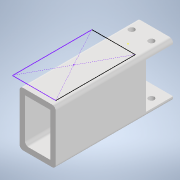
# Autodesk Inventor part: SUCTION_EXTENSION1
Saved by Autodesk Inventor 2021 (Build 250183000, 183)
## iProperties
Created: 2023-03-20
Part Number: SUCTION_EXTENSION1
Material: Generic
Document SubType Name: Modeling
Designer: mahmo
Density: 1 g/cm^3
Appearance: Default
Author: mahmo
Autodesk Inventor part; units mm, degrees
ref_plane "YZ Plane" through (0, 0, 0) normal (1, 0, 0) x (0, 1, 0)
ref_plane "XZ Plane" through (0, 0, 0) normal (0, 1, 0) x (-1, 0, 0)
ref_plane "XY Plane" through (0, 0, 0) normal (0, 0, 1) x (1, 0, 0)
sketch "Sketch1" plane through (0, 0, 0) normal (0, 0, 1) x (1, 0, 0)
  line L0 (-10, 15) -> (10, 15)
  line L1 (10, 15) -> (10, -15)
  line L2 (10, -15) -> (-10, -15)
  line L3 (-10, -15) -> (-10, 15)
  line L4 (-10, 15) -> (10, -15) construction
  line L5 (10, 15) -> (-10, -15) construction
  point P0 (0, 0)
  dimension "d0" = 20
  dimension "d1" = 30
  constraints: 12 end point, 2 midpoint, 2 parallel, 1 horizontal, 1 perpendicular
  measures "d0" distance of L1.end L2.end
  measures "d1" distance of L0.end L1.end
extrude "Extrusion1" add sketch "Sketch1" along normal blind 50
shell "Shell1" thickness 3 removed faces 1 at (-3.3333, 5, 50)
sketch "Sketch2" plane through (-10, 15, 0) normal (0, 1, 0) x (1, 0, 0)
  line L0 (3, -3) -> (17, -3) projected
  line L1 (-7, -47) -> (17, -47)
  line L2 (17, -47) -> (17, -3)
  line L3 (17, -3) -> (-7, -3)
  line L4 (-7, -3) -> (-7, -47)
  line L5 (-7, -47) -> (17, -3) construction
  line L6 (17, -47) -> (-7, -3) construction
  point P0 (10, 0)
  point P1 (5, -25)
  constraints: 12 end point, 2 midpoint, 2 parallel, 1 horizontal, 1 perpendicular
sketch "Sketch3" plane through (0, 0, 0) normal (0, 0, -1) x (-1, 0, 0)
  line L0 (-10, 15) -> (10, 15) projected
  line L1 (10, 15) -> (10, -15) projected
  line L2 (-10, 15) -> (10, 15)
  line L3 (10, 15) -> (10, 12.5)
  line L4 (10, 12.5) -> (-10, 12.5)
  line L5 (-10, 12.5) -> (-10, 15)
  line L6 (-10, -15) -> (-10, 15) projected
  line L7 (10, -15) -> (-10, -15)
  line L8 (-10, -15) -> (-10, -12.5)
  line L9 (-10, -12.5) -> (10, -12.5)
  line L10 (10, -12.5) -> (10, -15)
  point P0 (0, 0)
  point P1 (10, -12.5)
  dimension "d5" = 2.5
  dimension "d6" = 2.5
  constraints: 16 end point, 4 parallel, 2 horizontal, 2 perpendicular, 2 point on line
  measures "d5" distance of L2.end L3.end
  measures "d6" distance of L7.end L8.end
extrude "Extrusion2" add sketch "Sketch3" along normal blind 15 contours L0 L1 L4 L5 | L9 L1 L7 L6
sketch "Sketch4" plane through (-10, 15, 50) normal (0, 1, 0) x (1, 0, 0)
  point P0 (10, 50)
sketch "Sketch6" plane through (-10, -15, 50) normal (0, -1, 0) x (1, 0, 0)
  circle A0 centre (4.0698, -58) radius 1.6 projected
  circle A1 centre (15, -58) radius 1.6 projected
  point P0 (10, -50)
extrude "Extrusion4" cut sketch "Sketch6" against normal through all
fillet "Fillet1" radius 2 4 edges at (-7, -12, 26.5) (10, -15, 17.5) (-10, 15, 17.5) (10, 15, 17.5)
fillet "Fillet2" radius 2 1 edges at (-10, -15, 17.5)
sketch "Sketch7" plane through (8, -15, -15) normal (0, -1, 0) x (1, 0, 0)
  circle A0 centre (-8, 25.9391) radius 2.5
  point P0 (-8, 15)
  dimension "d17" = 5
  constraints: 1 centre point
  measures "d17" diameter of A0
extrude "Extrusion5" cut sketch "Sketch7" against normal blind 10
sketch "Sketch8" plane through (0, 0, 50) normal (0, 0, 1) x (1, 0, 0)
  line L0 (-10, 12.5) -> (-10, -12.5) projected
  line L1 (10, -0.5) -> (-10, -0.5)
  line L2 (-10, -0.5) -> (-10, 0.5)
  line L3 (-10, 0.5) -> (10, 0.5)
  line L4 (10, 0.5) -> (10, -0.5)
  line L5 (10, -0.5) -> (-10, 0.5) construction
  line L6 (-10, -0.5) -> (10, 0.5) construction
  point P0 (0, 0)
  dimension "d20" = 1
  constraints: 12 end point, 2 midpoint, 2 parallel, 1 horizontal, 1 perpendicular, 1 point on line
  measures "d20" distance of L1.end L2.end
extrude "Extrusion6" cut sketch "Sketch8" against normal blind 30
sketch "Sketch9" plane through (0, 0, 50) normal (0, 0, 1) x (1, 0, 0)
  line L0 (-7, 0.5) -> (-3.9859, 12)
  line L1 (-7, 12) -> (7, 12) projected
  line L2 (-3.9859, 12) -> (2.913, 12)
  line L3 (7, 0.5) -> (2.913, 12)
  line L4 (7, -0.5) -> (2.3967, -12.0157)
  line L5 (2.3967, -12.0157) -> (-2.9074, -12.0157)
  line L6 (7, -12) -> (7, 12) projected
  line L7 (-7, -10) -> (-7, -0.5) projected
  line L8 (-2.9074, -12.0157) -> (-7, -0.5)
  line L9 (-7, -0.5) -> (7, -0.5)
  line L10 (10, -12.5) -> (10, 12.5) projected
  line L11 (7, 0.5) -> (-7, 0.5)
  line L12 (10, 12.5) -> (-10, 12.5) projected
  line L13 (7, -12) -> (-5, -12) projected
  arc A0 (-7, -10) -> (-5, -12) centre (-5, -10) ccw projected
  line L14 (-7, 0.5) -> (-7, 12) projected
  point P0 (0, 0)
  point P1 (2.403, -12)
  point P2 (-2.913, -12)
  constraints: 16 end point, 2 parallel, 2 perpendicular, 2 point on line
extrude "Extrusion7" add sketch "Sketch9" against normal blind 30 contours L14 L1 L0 | L3 L1 L6 | L6 L13 L4 | L8 L13 A0 L7
sketch "Sketch10" plane through (10, -12.5, 0) normal (1, 0, 0) x (0, 0, -1)
  line L0 (-20, 12) -> (-50, 12) projected
  line L1 (-50, 12) -> (-43.1699, 12)
  line L2 (-43.1699, 12) -> (-43.1699, 9.596)
  line L3 (-43.1699, 9.596) -> (-50, 9.596)
  line L4 (-50, 9.596) -> (-50, 12)
  line L5 (-50, 13) -> (-43.1699, 13)
  line L6 (-43.1699, 13) -> (-43.1699, 14.6143)
  line L7 (-43.1699, 14.6143) -> (-50, 14.6143)
  line L8 (-50, 14.6143) -> (-50, 13)
  point P0 (0, 12.5)
  constraints: 16 end point, 4 parallel, 2 horizontal, 2 perpendicular, 1 point on line
extrude "Extrusion8" add sketch "Sketch10" along normal blind 5
sketch "Sketch11" plane through (10, -2.904, 43.1699) normal (0, -1, 0) x (1, 0, 0)
  circle A0 centre (2.6177, 3.2863) radius 1.5609
  point P0 (-10, -43.1699)
  constraints: 1 centre point
extrude "Extrusion9" cut sketch "Sketch11" against normal blind 6.25
mirror "Mirror1" about plane through (0, 0, 0) normal (1, 0, 0) of "Extrusion8", "Extrusion9"
body "Solid1"
